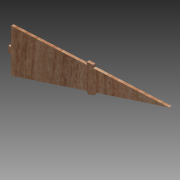
# Autodesk Inventor part: Star Side Out
Saved by Autodesk Inventor 2015 (Build 190159000, 159)
## iProperties
Created: 2018-03-07
Part Number: Star Side Out
Material: Wood (Birch)
Document SubType Name: Modeling
Designer: Administrator
Density: 0.55 g/cm^3
Appearance: Birch - Natural Polished
Mass: 9.05421 g
Surface Area: 118.577 cm^2
Volume: 16.4622 cm^3
Author: Administrator
Autodesk Inventor part; units mm, degrees
ref_plane "YZ Plane" through (0, 0, 0) normal (1, 0, 0) x (0, 1, 0)
ref_plane "XZ Plane" through (0, 0, 0) normal (0, 1, 0) x (-1, 0, 0)
ref_plane "XY Plane" through (0, 0, 0) normal (0, 0, 1) x (1, 0, 0)
sketch "Sketch1" plane through (0, 0, 0) normal (0, 0, 1) x (1, 0, 0)
  line L0 (0, 0) -> (0, 52.9336)
  line L1 (0, 52.9336) -> (193.1614, 63.023)
  line L2 (193.1614, 63.023) -> (0, 0)
  dimension "d0" = 52.9336
  dimension "d34" = 15.08
  dimension "d48" = 92.99
  constraints: 6 end point, 1 vertical
  measures "d0" distance of L0.start L0.end
  measures "d34" angle of L2 L1
  measures "d48" angle of L0 L1
extrude "Extrusion1" add sketch "Sketch1" along normal blind 3.175
sketch "Sketch5" plane through (0, 0, 3.175) normal (0, 0, 1) x (1, 0, 0)
  line L0 (0, 52.9336) -> (0, 0) projected
  line L1 (193.1614, 63.023) -> (0, 52.9336) projected
  line L2 (0, 30.2768) -> (-3.175, 30.2768)
  line L3 (-3.175, 30.2768) -> (-3.175, 22.6568)
  line L4 (-3.175, 22.6568) -> (0, 22.6568)
  line L5 (0, 22.6568) -> (0, 30.2768)
  line L6 (100.3855, 58.177) -> (100.2199, 61.3477)
  line L7 (100.2199, 61.3477) -> (92.6103, 60.9502)
  line L8 (92.6103, 60.9502) -> (92.7759, 57.7795)
  line L9 (92.7759, 57.7795) -> (100.3855, 58.177)
  line L10 (0, 0) -> (193.1614, 63.023) projected
  line L11 (100.2028, 32.6933) -> (101.1876, 29.6749)
  line L12 (101.1876, 29.6749) -> (93.9434, 27.3113)
  line L13 (93.9434, 27.3113) -> (92.9586, 30.3297)
  line L14 (92.9586, 30.3297) -> (100.2028, 32.6933)
  point P0 (0, 26.4668)
  point P1 (96.5807, 57.9783)
  point P2 (96.5807, 31.5115)
  dimension "d36" = 7.62
  dimension "d37" = 3.81
  dimension "d38" = 3.175
  dimension "d39" = 3.81
  dimension "d40" = 7.62
  dimension "d41" = 3.175
  dimension "d42" = 3.81
  dimension "d44" = 7.62
  dimension "d45" = 3.175
  constraints: 24 end point, 6 point on line, 5 parallel, 5 perpendicular, 3 collinear, 3 midpoint, 1 horizontal
  measures "d36" distance between parallel lines of L4 L2
  measures "d37" distance from line of L2 point (0, 26.467)
  measures "d38" distance between parallel lines of L0 L3
  measures "d39" distance from line of L6 point (96.581, 57.978)
  measures "d40" distance between parallel lines of L6 L8
  measures "d41" distance between parallel lines of L1 L7
  measures "d42" distance from line of L11 point (96.581, 31.511)
  measures "d44" distance between parallel lines of L11 L13
  measures "d45" distance between parallel lines of L14 L12
extrude "Extrusion5" add sketch "Sketch5" against normal blind 3.175 contours L0 L4 L3 L2 | L8 L7 L6 L1 | L10 L11 L12 L13
sketch "Sketch6" plane through (0, 0, 3.175) normal (0, 0, 1) x (1, 0, 0)
  line L0 (0, 0) -> (0, 22.6568)
  line L1 (0, 22.6568) -> (-3.175, 22.6568)
  line L2 (-3.175, 22.6568) -> (-3.175, 30.2768)
  line L3 (-3.175, 22.6568) -> (-3.175, 30.2768) projected
  line L4 (-3.175, 30.2768) -> (0, 30.2768)
  line L5 (0, 30.2768) -> (0, 52.9336)
  line L6 (0, 30.2768) -> (0, 52.9336) projected
  line L7 (0, 52.9336) -> (92.7759, 57.7795)
  line L8 (92.7759, 57.7795) -> (0, 52.9336) projected
  line L9 (92.7759, 57.7795) -> (92.6103, 60.9502)
  line L10 (92.6103, 60.9502) -> (100.2199, 61.3477)
  line L11 (92.6103, 60.9502) -> (100.2199, 61.3477) projected
  line L12 (100.2199, 61.3477) -> (100.3855, 58.177)
  line L13 (100.3855, 58.177) -> (193.1614, 63.023)
  line L14 (100.3855, 58.177) -> (193.1614, 63.023) projected
  line L15 (193.1614, 63.023) -> (100.2028, 32.6933)
  line L16 (101.1876, 29.6749) -> (93.9434, 27.3113) projected
  line L17 (100.2028, 32.6933) -> (101.1876, 29.6749)
  line L18 (101.1876, 29.6749) -> (93.9434, 27.3113)
  line L19 (93.9434, 27.3113) -> (92.9586, 30.3297)
  line L20 (92.9586, 30.3297) -> (0, 0)
  line L21 (92.9586, 30.3297) -> (0, 0) projected
  constraints: 30 end point, 7 perpendicular, 6 collinear, 1 parallel, 1 vertical
body "Solid1"
